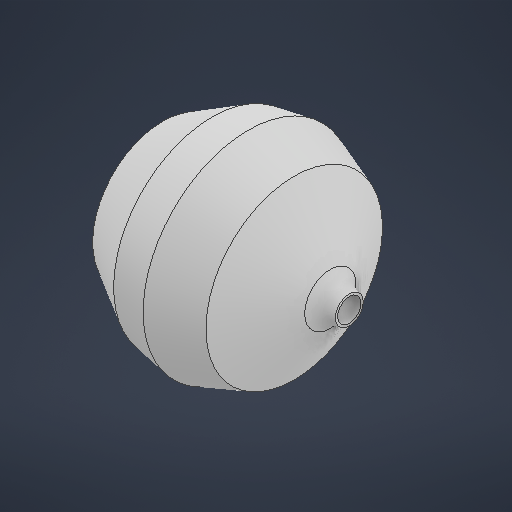
# Autodesk Inventor part: cola
Saved by Autodesk Inventor 2026.2 (Build 302298000, 298)
## iProperties
Created: 2026-05-21
Part Number: cola
Material: Generic
Document SubType Name: Modeling
Designer: juand
Density: 1 g/cm^3
Appearance: Default
Author: juand
Autodesk Inventor part; units mm, degrees
ref_plane "YZ Plane" through (0, 0, 0) normal (1, 0, 0) x (0, 1, 0)
ref_plane "XZ Plane" through (0, 0, 0) normal (0, 1, 0) x (-1, 0, 0)
ref_plane "XY Plane" through (0, 0, 0) normal (0, 0, 1) x (1, 0, 0)
sketch "Sketch3" plane through (0, 0, 0) normal (0, 0, 1) x (1, 0, 0)
  line L0 (0, 0) -> (-80, 0)
  line L1 (0, 0) -> (0, 5)
  arc A0 (0, 5) -> (-5, 0) centre (0, 0) ccw
  line L2 (0, 5) -> (0, 6)
  arc A1 (0, 6) -> (-6, 0) centre (0, 0) ccw
  line L3 (-4.2426, 4.2426) -> (-23.6271, 37.8176)
  line L4 (-23.6271, 37.8176) -> (-43.3607, 45)
  line L5 (-43.3607, 45) -> (-58.7057, 42.2943)
  line L6 (-58.7057, 42.2943) -> (-80, 30)
  line L7 (-80, 30) -> (-80, 0)
  line L8 (-79, 0) -> (-79, 29.4226)
  line L9 (-79, 29.4226) -> (-58.3584, 41.3401)
  line L10 (-58.3584, 41.3401) -> (-43.4509, 43.9687)
  line L11 (-43.4509, 43.9687) -> (-24.3112, 37.0024)
  line L12 (-24.3112, 37.0024) -> (-4.9258, 3.4259)
  dimension "d14" = 5
  dimension "d15" = 1
  dimension "d16" = 90
  dimension "d17" = 120
  dimension "d18" = 160
  dimension "d19" = 150
  dimension "d20" = 40
  dimension "d21" = 30
  dimension "d22" = 80
  dimension "d23" = 21
  dimension "d24" = 1
  constraints: 26 end point, 6 point on circle, 3 point on line, 3 vertical, 2 centre point, 2 coincident, 1 horizontal, 4 other
  measures "d14" radius of A0
  measures "d15" radial gap between concentric circles of A1 A0
  measures "d16" diameter of L4.end L0
  measures "d17" angle of L7 L6
  measures "d18" angle of L6 L5
  measures "d19" angle of L4 L5
  measures "d20" angle of L3 L4
  measures "d21" distance of L6.end L0.end
  measures "d22" distance of L0.start L0.end
  measures "d23" distance of L3.end L4.end
  measures "d24" distance between parallel lines of L12 L3
revolve "Revolution2" add sketch "Sketch3" angle 360 about axis through (0, 0, 0) along (-1, 0, 0) contours L0 A1 L2 A0 | L0 L7 L6 L5 L4 L3 A1 L12 L11 L10 L9 L8
fillet "Fillet2" radius 10 1 edges at (-4.2426, -4.2426, 0)
body "Solid2"
